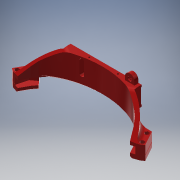
# Autodesk Inventor part: clamp_r
Saved by Autodesk Inventor 2017 (Build 210142000, 142)
## iProperties
Created: 2016-11-21
Part Number: clamp_r
Material: PC/ABS Plastic
Document SubType Name: Modeling
Designer: Ali
Density: 0.357273 g/cm^3
Appearance: Smooth - Red
Author: Ali
Autodesk Inventor part; units mm, degrees
sketch "Sketch1" plane through (0, 0, 0) normal (0, 0, 1) x (1, 0, 0)
  arc A0 (-5.3802, 56.637) -> (-102.6346, 44.8571) centre (-44.3802, -28.7347) ccw projected
  arc A1 (-102.6346, 44.8571) -> (-108.3066, 14.3732) centre (55.6325, -0.3603) ccw projected
  line L0 (-108.3066, 14.3732) -> (-107.3533, 6.1304) projected
  line L1 (-107.3533, 6.1304) -> (-107.3505, 6.0507) projected
  arc A2 (-107.3505, 6.0507) -> (-89.5835, -54.6922) centre (20.8962, 10.5923) ccw projected
  arc A3 (-89.5835, -54.6922) -> (-67.6974, -85.6874) centre (112.0298, 64.4449) ccw projected
  line L2 (-67.6974, -85.6874) -> (-66.8062, -86.7543) projected
  arc A4 (-66.8062, -86.7543) -> (-66.6302, -85.4767) centre (-71.3562, -85.4767) ccw projected
  arc A5 (-66.6302, -85.4767) -> (-74.3323, -73.8524) centre (-117.1754, -110.6039) ccw projected
  line L3 (-88.3802, -53.9767) -> (-74.3323, -73.8524) projected
  arc A6 (-105.1302, -3.9767) -> (-88.3802, -53.9767) centre (19.6205, 10.0092) ccw projected
  arc A7 (-104.1051, 25.3968) -> (-105.1302, -3.9767) centre (-5.1046, 7.2372) ccw projected
  spline S0 degree 4 poles (-44.3802, 62.2233) (-60.9817, 62.2233) (-84.9184, 55.4182) (-96.719, 46.0233) (-101.8787, 37.5346) (-104.1051, 25.3968) knots 1 1 1 1 1 2 3 3 3 3 3 projected
  spline S1 degree 4 poles (-44.3802, 62.2233) (-27.7787, 62.2233) (-3.8419, 55.4182) (7.9586, 46.0233) (13.1183, 37.5346) (15.3447, 25.3968) knots 1 1 1 1 1 2 3 3 3 3 3 projected
  arc A8 (16.3698, -3.9767) -> (15.3447, 25.3968) centre (-83.6558, 7.2372) ccw projected
  arc A9 (-0.3802, -53.9767) -> (16.3698, -3.9767) centre (-108.3809, 10.0092) ccw projected
  line L4 (-0.3802, -53.9767) -> (-14.428, -73.8524) projected
  arc A10 (-14.428, -73.8524) -> (-22.1302, -85.4767) centre (28.415, -110.6039) ccw projected
  arc A11 (-22.1302, -85.4767) -> (-21.9542, -86.7543) centre (-17.4041, -85.4767) ccw projected
  line L5 (-21.9542, -86.7543) -> (-21.063, -85.6874) projected
  arc A12 (-21.063, -85.6874) -> (0.8231, -54.6922) centre (-200.7901, 64.4449) ccw projected
  arc A13 (0.8231, -54.6922) -> (18.5901, 6.0507) centre (-109.6566, 10.5923) ccw projected
  line L6 (18.5901, 6.0507) -> (18.593, 6.1304) projected
  line L7 (18.593, 6.1304) -> (19.5462, 14.3732) projected
  arc A14 (19.5462, 14.3732) -> (13.8743, 44.8571) centre (-144.3928, -0.3603) ccw projected
  arc A15 (13.8743, 44.8571) -> (6.6198, 50.0583) centre (-44.3802, -28.7347) ccw projected
  line L8 (6.6198, 61.5233) -> (6.6198, 50.0583) projected
  line L9 (-5.3802, 61.5233) -> (6.6198, 61.5233) projected
  line L10 (-5.3802, 56.637) -> (-5.3802, 61.5233) projected
  line L11 (14.5194, 32.9809) -> (9.6506, 41.7615)
  line L12 (10.1861, 51.0026) -> (12.6488, 53.6391)
  line L13 (12.6488, 53.6391) -> (16.7857, 53.6391)
  line L14 (16.7857, 53.6391) -> (25.5146, 37.8973)
  line L15 (22.0832, 35.5866) -> (14.5194, 32.9809)
  line L16 (22.0832, 35.5866) -> (25.5146, 37.8973)
  line L17 (22.0832, 35.5866) -> (12.6488, 53.6391) construction
  line L18 (9.6506, 41.7615) -> (6.0073, 46.5287)
  line L19 (6.0073, 46.5287) -> (10.1861, 51.0026)
  line L20 (16.6197, 32.5233) -> (16.8713, 18.1048) projected
  line L21 (16.8878, 32.528) -> (16.6197, 32.5233) projected
  line L22 (16.8878, 32.528) -> (18.6194, 32.5582) projected
  line L23 (18.871, 18.1397) -> (18.6194, 32.5582) projected
  line L24 (18.871, 18.1397) -> (16.8713, 18.1048) projected
  line L25 (6.0073, 46.5287) -> (14.5194, 32.9809) construction
  point P0 (0, 0)
  dimension "d1" = 8
  dimension "d2" = 12
  dimension "d5" = 18
  dimension "d8" = 100
  dimension "d9" = 16
  dimension "d10" = 6
  constraints: 21 end point, 1 collinear, 1 equal length, 1 horizontal, 1 other
  measures "d1" distance of L15.start L11.start
  measures "d2" distance between parallel lines of L11 L14
  measures "d5" distance of L13.end L14.end
  measures "d8" angle of L15 L11
  measures "d9" distance of L18.end L11.start
  measures "d10" distance of L11.end L18.end
extrude "Extrusion1" add sketch "Sketch1" along normal blind 3 contours L19 L12 L13 L14 L16 L15 A14 A15 | A15 A14 L15 L11 L18 L19
sketch "Sketch2" plane through (0, 0, 0) normal (0, 0, -1) x (-1, 0, 0)
  line L0 (-14.5194, 32.9809) -> (-9.6506, 41.7615) projected
  line L1 (-9.6506, 41.7615) -> (-6.0073, 46.5287) projected
  line L2 (-6.0073, 46.5287) -> (-12.6488, 53.6391) projected
  line L3 (-12.6488, 53.6391) -> (-16.7857, 53.6391) projected
  line L4 (-16.7857, 53.6391) -> (-25.5146, 37.8973) projected
  line L5 (-25.5146, 37.8973) -> (-22.0832, 35.5866) projected
  line L6 (-22.0832, 35.5866) -> (-14.5194, 32.9809) projected
  line L7 (-6.0073, 46.5287) -> (-12.6488, 53.6391) projected
  line L8 (-12.6488, 53.6391) -> (-16.7857, 53.6391) projected
  line L9 (-9.328, 50.0839) -> (-12.6488, 53.6391)
  line L10 (-22.0832, 35.5866) -> (-14.5194, 32.9809) projected
  line L11 (-18.7662, 34.4439) -> (-22.0832, 35.5866)
  line L12 (-18.7662, 34.4439) -> (-15.745, 46.1362)
  line L13 (-12.6488, 53.6391) -> (-6.0073, 46.5287) projected
  line L14 (-9.7584, 50.5447) -> (-15.745, 46.1362)
  point P0 (0, 0)
  constraints: 8 end point, 2 point on line, 1 collinear, 1 midpoint
extrude "Extrusion2" add sketch "Sketch2" along normal blind 6.5 contours L6 L5 L4 L3 L2 L14 L12
sketch "Sketch3" plane through (0, 0, -6.5) normal (0, 0, -1) x (-1, 0, 0)
  line L0 (-9.6506, 41.7615) -> (-14.5194, 32.9809) projected
  line L1 (-14.5194, 32.9809) -> (-22.0832, 35.5866) projected
  line L2 (-22.0832, 35.5866) -> (-25.5146, 37.8973) projected
  line L3 (-25.5146, 37.8973) -> (-16.7857, 53.6391) projected
  line L4 (-16.7857, 53.6391) -> (-12.6488, 53.6391) projected
  line L5 (-12.6488, 53.6391) -> (-6.0073, 46.5287) projected
  line L6 (-6.0073, 46.5287) -> (-9.6506, 41.7615) projected
  point P0 (0, 0)
extrude "Extrusion3" add sketch "Sketch3" along normal blind 5 separate body
chamfer "Chamfer1" distance 1.5 angle 45 2 edges at (12.085, 37.3712, -11.5) (7.8289, 44.1451, -11.5)
sketch "Sketch4" plane through (0, 0, -11.5) normal (0, 0, -1) x (-1, 0, 0)
  line L0 (-7.0457, 47.6404) -> (-10.9091, 42.585) projected
  line L1 (-7.0457, 47.6404) -> (-12.6488, 53.6391) projected
  line L2 (-12.6488, 53.6391) -> (-16.7857, 53.6391) projected
  line L3 (-16.7857, 53.6391) -> (-25.5146, 37.8973) projected
  line L4 (-25.5146, 37.8973) -> (-22.0832, 35.5866) projected
  line L5 (-22.0832, 35.5866) -> (-15.9595, 33.477) projected
  line L6 (-10.9091, 42.585) -> (-15.9595, 33.477) projected
  point P0 (0, 0)
  point P1 (-15.5734, 49.6391)
  point P2 (-21.3927, 39.1446)
  dimension "d19" = 12
  dimension "d20" = 4
  dimension "d21" = 3
  dimension "d22" = 3
  measures "d19" distance of point (-21.393, 39.145) point (-15.573, 49.639)
  measures "d20" distance from line of L2 point (-15.573, 49.639)
  measures "d21" distance from line of L3 point (-15.573, 49.639)
  measures "d22" distance from line of point (-21.393, 39.145) L3
hole "Hole1" at (15.5734, 49.6391, -11.5) at (21.3927, 39.1446, -11.5) direction (0, 0, 1) diameter 2.2 end through all bodies 2
sketch "Sketch5" plane through (0, 0, -6.5) normal (0, 0, -1) x (-1, 0, 0)
  circle A0 centre (-21.3927, 39.1446) radius 1.1 projected
  circle A1 centre (-15.5734, 49.6391) radius 1.1 projected
  point P0 (0, 0)
hole "Hole2" at (21.3927, 39.1446, -6.5) at (15.5734, 49.6391, -6.5) direction (0, 0, 1) diameter 2.2 end through all bodies 1
ref_plane "Work Plane1" through (0, 0, 0) normal (0, 0, 1) x (1, 0, 0)
sketch "Sketch6" plane through (0, 0, 0) normal (0, 0, 1) x (1, 0, 0)
  arc A0 (-5.3802, 56.637) -> (-102.6346, 44.8571) centre (-44.3802, -28.7347) ccw projected
  arc A1 (-102.6346, 44.8571) -> (-108.3066, 14.3732) centre (55.6325, -0.3603) ccw projected
  line L0 (-108.3066, 14.3732) -> (-107.3533, 6.1304) projected
  line L1 (-107.3533, 6.1304) -> (-107.3505, 6.0507) projected
  arc A2 (-107.3505, 6.0507) -> (-89.5835, -54.6922) centre (20.8962, 10.5923) ccw projected
  arc A3 (-89.5835, -54.6922) -> (-67.6974, -85.6874) centre (112.0298, 64.4449) ccw projected
  line L2 (-67.6974, -85.6874) -> (-66.8062, -86.7543) projected
  arc A4 (-66.8062, -86.7543) -> (-66.6302, -85.4767) centre (-71.3562, -85.4767) ccw projected
  arc A5 (-66.6302, -85.4767) -> (-74.3323, -73.8524) centre (-117.1754, -110.6039) ccw projected
  line L3 (-88.3802, -53.9767) -> (-74.3323, -73.8524) projected
  arc A6 (-105.1302, -3.9767) -> (-88.3802, -53.9767) centre (19.6205, 10.0092) ccw projected
  arc A7 (-104.1051, 25.3968) -> (-105.1302, -3.9767) centre (-5.1046, 7.2372) ccw projected
  spline S0 degree 4 poles (-44.3802, 62.2233) (-60.9817, 62.2233) (-84.9184, 55.4182) (-96.719, 46.0233) (-101.8787, 37.5346) (-104.1051, 25.3968) knots 1 1 1 1 1 2 3 3 3 3 3 projected
  spline S1 degree 4 poles (-44.3802, 62.2233) (-27.7787, 62.2233) (-3.8419, 55.4182) (7.9586, 46.0233) (13.1183, 37.5346) (15.3447, 25.3968) knots 1 1 1 1 1 2 3 3 3 3 3 projected
  arc A8 (16.3698, -3.9767) -> (15.3447, 25.3968) centre (-83.6558, 7.2372) ccw projected
  arc A9 (-0.3802, -53.9767) -> (16.3698, -3.9767) centre (-108.3809, 10.0092) ccw projected
  line L4 (-0.3802, -53.9767) -> (-14.428, -73.8524) projected
  arc A10 (-14.428, -73.8524) -> (-22.1302, -85.4767) centre (28.415, -110.6039) ccw projected
  arc A11 (-22.1302, -85.4767) -> (-21.9542, -86.7543) centre (-17.4041, -85.4767) ccw projected
  line L5 (-21.9542, -86.7543) -> (-21.063, -85.6874) projected
  arc A12 (-21.063, -85.6874) -> (0.8231, -54.6922) centre (-200.7901, 64.4449) ccw projected
  arc A13 (0.8231, -54.6922) -> (18.5901, 6.0507) centre (-109.6566, 10.5923) ccw projected
  line L6 (18.5901, 6.0507) -> (18.593, 6.1304) projected
  line L7 (18.593, 6.1304) -> (19.5462, 14.3732) projected
  arc A14 (19.5462, 14.3732) -> (13.8743, 44.8571) centre (-144.3928, -0.3603) ccw projected
  arc A15 (13.8743, 44.8571) -> (6.6198, 50.0583) centre (-44.3802, -28.7347) ccw projected
  line L8 (6.6198, 61.5233) -> (6.6198, 50.0583) projected
  line L9 (-5.3802, 61.5233) -> (6.6198, 61.5233) projected
  line L10 (-5.3802, 56.637) -> (-5.3802, 61.5233) projected
  line L11 (-44.3802, 62.2233) -> (-44.3802, 62.8011) construction
  circle A16 centre (21.3927, 39.1446) radius 1.1 projected
  circle A17 centre (15.5734, 49.6391) radius 1.1 projected
  line L12 (9.6506, 41.7615) -> (14.5194, 32.9809) projected
  line L13 (14.5194, 32.9809) -> (22.0832, 35.5866) projected
  line L14 (22.0832, 35.5866) -> (25.5146, 37.8973) projected
  line L15 (25.5146, 37.8973) -> (16.7857, 53.6391) projected
  line L16 (16.7857, 53.6391) -> (12.6488, 53.6391) projected
  line L17 (12.6488, 53.6391) -> (6.0073, 46.5287) projected
  line L18 (6.0073, 46.5287) -> (9.6506, 41.7615) projected
  spline S2 degree 3 poles (6.0073, 46.5287) (-6.3628, 57.3321) (-25.7237, 62.8011) (-44.3802, 62.8011) knots 0 0 0 0 1 1 1 1
  line L19 (-44.3802, 62.8011) -> (-44.3802, 66.8011)
  line L20 (16.7857, 53.6391) -> (12.6488, 53.6391) projected
  line L21 (12.6488, 53.6391) -> (0.9642, 53.6391) construction
  line L22 (0.9642, 53.6391) -> (-13.174, 64.4449) construction
  line L23 (-13.174, 64.4449) -> (-32.5316, 66.8011) construction
  line L24 (-32.5316, 66.8011) -> (-44.3802, 66.8011) construction
  spline S3 degree 4 poles (12.6488, 53.6391) (0.9642, 53.6391) (-13.174, 64.4449) (-32.5316, 66.8011) (-44.3802, 66.8011) knots 1 1 1 1 1 2 2 2 2 2
  point P0 (0, 0)
  point P1 (-15.8694, 58.4105)
  dimension "d38" = 4
  constraints: 4 end point, 4 vertical, 1 collinear, 6 other
  measures "d38" distance of L11.end L19.end
extrude "Extrusion4" add sketch "Sketch6" along normal up to surface (3 mm away) contours L10 S3 L8 A15 L17 S2 L19 A0 | A0 L19 S3 L10 | S3 L17 A15 L8 bodies 1
sketch "Sketch7" plane through (0, 0, 3) normal (0, 0, 1) x (1, 0, 0)
  circle A0 centre (21.3927, 39.1446) radius 1.1 projected
  circle A1 centre (15.5734, 49.6391) radius 1.1 projected
  line L0 (9.6506, 41.7615) -> (14.5194, 32.9809) projected
  line L1 (14.5194, 32.9809) -> (22.0832, 35.5866) projected
  line L2 (22.0832, 35.5866) -> (25.5146, 37.8973) projected
  line L3 (25.5146, 37.8973) -> (16.7857, 53.6391) projected
  line L4 (16.7857, 53.6391) -> (12.6488, 53.6391) projected
  spline S0 degree 4 poles (-44.3802, 66.8011) (-32.5316, 66.8011) (-13.174, 64.4449) (0.9642, 53.6391) (12.6488, 53.6391) knots 0 0 0 0 0 1 1 1 1 1 projected
  line L5 (-44.3802, 62.8011) -> (-44.3802, 66.8011) projected
  spline S1 degree 3 poles (6.0073, 46.5287) (-6.3628, 57.3321) (-25.7237, 62.8011) (-44.3802, 62.8011) knots 0 0 0 0 1 1 1 1 projected
  line L6 (6.0073, 46.5287) -> (9.6506, 41.7615) projected
  line L7 (14.5194, 32.9809) -> (22.0832, 35.5866) projected
  arc A2 (18.7914, 34.4526) -> (-7.163, 59.1735) centre (-22.4149, 17.1754) ccw
  line L8 (-7.163, 59.1735) -> (-7.163, 66.8011)
  line L9 (-44.3802, 66.8011) -> (-44.3802, 62.8011) projected
  line L10 (-7.163, 66.8011) -> (-44.3802, 66.8011)
  point P0 (0, 0)
  constraints: 4 end point, 2 point on circle, 1 centre point, 1 perpendicular, 1 point on line, 1 vertical, 4 other
extrude "Extrusion5" add sketch "Sketch7" along normal blind 24 contours L6 S1 L5 S0 A2 L1 L0 | S0 L10 L8 bodies 1
sketch "Sketch13" plane through (0, 0, 3) normal (0, 0, -1) x (-1, 0, 0)
  spline S0 degree 4 poles (44.3802, 66.8011) (36.9623, 66.8011) (26.6014, 65.8776) (16.4206, 62.5354) (7.163, 59.1735) knots 0 0 0 0 0 1 1 1 1 1 projected
  line L0 (7.163, 66.8011) -> (44.3802, 66.8011) projected
  line L1 (7.163, 59.1735) -> (7.163, 66.8011) projected
  point P0 (0, 0)
  constraints: 1 other
extrude "Extrusion10" cut sketch "Sketch13" against normal blind 4 bodies 1
sketch "Sketch8" plane through (16.7857, 53.6391, 3) normal (0.8745473, 0.4849403, 0) x (0, 0, -1)
  line L0 (0, -17.7522) -> (-24, -17.7522) projected
  line L1 (-24, 16.4538) -> (-24, 23.1244) projected
  line L2 (0, -17.7522) -> (-24, 16.4538)
  line L3 (-24, -17.7522) -> (-24, 16.4538)
  point P0 (3, -38.7699)
  constraints: 4 end point
extrude "Extrusion6" cut sketch "Sketch8" against normal through all bodies 1
sketch "Sketch15" plane through (0, 0, 3) normal (0, 0, 1) x (1, 0, 0)
  line L0 (25.5146, 37.8973) -> (16.7857, 53.6391) projected
  line L1 (16.7857, 53.6391) -> (12.6488, 53.6391) projected
  arc A0 (18.7914, 34.4526) -> (-7.163, 59.1735) centre (-22.4149, 17.1754) ccw projected
  line L2 (18.7914, 34.4526) -> (22.0832, 35.5866) projected
  line L3 (22.0832, 35.5866) -> (25.5146, 37.8973) projected
  circle A1 centre (21.3927, 39.1446) radius 1.1 projected
  circle A2 centre (15.5734, 49.6391) radius 1.1 projected
  line L4 (19.0547, 39.185) -> (20.2587, 41.1895)
  line L5 (20.2587, 41.1895) -> (22.5967, 41.149)
  line L6 (22.5967, 41.149) -> (23.7306, 39.1041)
  line L7 (23.7306, 39.1041) -> (22.5266, 37.0996)
  line L8 (22.5266, 37.0996) -> (20.1887, 37.1401)
  line L9 (20.1887, 37.1401) -> (19.0547, 39.185)
  circle A3 centre (15.5734, 49.6391) radius 1.1 projected
  line L10 (13.2355, 49.6796) -> (14.4395, 51.6841)
  line L11 (14.4395, 51.6841) -> (16.7774, 51.6436)
  line L12 (16.7774, 51.6436) -> (17.9113, 49.5987)
  line L13 (17.9113, 49.5987) -> (16.7073, 47.5942)
  line L14 (16.7073, 47.5942) -> (14.3694, 47.6347)
  line L15 (14.3694, 47.6347) -> (13.2355, 49.6796)
  line L16 (25.5146, 37.8973) -> (16.7857, 53.6391) projected
  point P0 (0, 0)
  dimension "d89" = 4.05
  dimension "d90" = 4.05
  constraints: 24 end point, 2 coincident, 2 parallel, 27 other
  measures "d89" distance between parallel lines of L4 L7
  measures "d90" distance between parallel lines of L13 L10
extrude "Extrusion11" cut sketch "Sketch15" against normal blind 4 bodies 1
mirror "Mirror1" about plane through (-44.3802, 66.8011, 0) normal (-1, 0, 0) of "Extrusion5", "Extrusion6", "Extrusion1", "Hole2", "Extrusion2", "Extrusion4", "Extrusion10", "Extrusion11" bodies 1
sketch "Sketch9" plane through (-7.163, 66.8011, 27) normal (0, 1, 0) x (1, 0, 0)
  line L0 (41.7828, 2) -> (-116.2172, 2)
  line L1 (-116.2172, 2) -> (-116.2172, 18)
  line L2 (-116.2172, 18) -> (41.7828, 18)
  line L3 (41.7828, 18) -> (41.7828, 2)
  line L4 (-74.4343, 20) -> (-74.4343, 0) projected
  line L5 (0, 0) -> (-74.4343, 0) projected
  line L6 (0, 20) -> (0, 0) projected
  line L7 (-37.2172, 24) -> (-37.2172, 0) construction
  line L8 (-74.4343, 24) -> (-37.2172, 24) projected
  line L9 (-56.7172, 16.2) -> (-56.7172, 3.8) construction
  line L10 (0, 20) -> (-37.2172, 20) projected
  line L11 (-37.2172, 20) -> (-74.4343, 20) projected
  point P0 (7.163, 27)
  point P1 (-37.2172, 2)
  dimension "d45" = 158
  dimension "d46" = 16
  dimension "d47" = 1.8
  dimension "d48" = 1.8
  dimension "d49" = 59.5
  dimension "d62" = 2
  constraints: 10 end point, 2 parallel, 1 horizontal, 1 midpoint, 1 perpendicular, 1 point on line, 1 vertical
  measures "d45" distance of L0.start L0.end
  measures "d46" distance of L0.end L1.end
  measures "d47" distance from line of L0 L9.end
  measures "d48" distance from line of L2 L9.start
  measures "d49" distance between parallel lines of L9 L1
  measures "d62" distance between parallel lines of L5 L0
hole "Hole3" at (-63.8802, 66.8011, 23.2) at (-63.8802, 66.8011, 10.8) direction (0, -1, 0) diameter 1.8 end through all bodies 1
ref_plane "Work Plane2" through (-7.163, 56.5511, 27) normal (0, 1, 0) x (1, 0, 0)
sketch "Sketch10" plane through (-7.163, 56.5511, 27) normal (0, 1, 0) x (1, 0, 0)
  spline S0 degree 2 poles (-56.7172, 2.9) (-58.276, 2.9) (-57.4966, 4.25) (-56.7172, 5.6) (-55.9377, 4.25) (-55.1583, 2.9) (-56.7172, 2.9) knots 0 0 0 0.333333 0.333333 0.666667 0.666667 1 1 1 weights 1 0.5 1 0.5 1 0.5 1 projected
  spline S1 degree 2 poles (-56.7172, 15.3) (-58.276, 15.3) (-57.4966, 16.65) (-56.7172, 18) (-55.9377, 16.65) (-55.1583, 15.3) (-56.7172, 15.3) knots 0 0 0 0.333333 0.333333 0.666667 0.666667 1 1 1 weights 1 0.5 1 0.5 1 0.5 1 projected
  circle A0 centre (-56.7172, 3.8) radius 0.9 projected
  circle A1 centre (-56.7172, 3.8) radius 2
  circle A2 centre (-56.7172, 16.2) radius 0.9 projected
  circle A3 centre (-56.7172, 16.2) radius 2
  line L0 (-54.7172, 16.2) -> (-54.7172, 3.8)
  line L1 (-58.7172, 3.8) -> (-58.7172, 16.2)
  point P0 (7.163, 27)
  dimension "d58" = 4
  dimension "d59" = 4
  constraints: 4 end point, 4 point on circle, 2 centre point, 2 coincident, 2 tangent, 2 vertical, 4 other
  measures "d58" diameter of A1
  measures "d59" diameter of A3
extrude "Extrusion7" cut sketch "Sketch10" along normal blind 8.6 bodies 1
sketch "Sketch11" plane through (-7.163, 66.8011, 27) normal (0, 1, 0) x (1, 0, 0)
  circle A0 centre (-56.7172, 3.8) radius 0.9 projected
  circle A1 centre (-56.7172, 16.2) radius 0.9 projected
  line L0 (-74.4343, 20) -> (-74.4343, 0) projected
  line L1 (0, 0) -> (-74.4343, 0) projected
  line L2 (0, 20) -> (0, 0) projected
  line L3 (0, 20) -> (0, 0) projected
  line L4 (0, 2) -> (-74.4343, 2)
  line L5 (-74.4343, 20) -> (-74.4343, 0) projected
  line L6 (-74.4343, 18) -> (0, 18)
  line L7 (-37.2172, 20) -> (-74.4343, 20) projected
  line L8 (0, 20) -> (-37.2172, 20) projected
  point P0 (7.163, 27)
  point P1 (0, 24)
  point P2 (-74.4343, 24)
  dimension "d63" = 2
  dimension "d78" = 16
  constraints: 4 end point, 4 point on line, 1 horizontal, 1 parallel
  measures "d63" distance between parallel lines of L1 L4
  measures "d78" distance between parallel lines of L4 L6
extrude "Extrusion8" cut sketch "Sketch11" against normal blind 0.5 contours A0 | A1 | L6 L2 L4 L0 bodies 1
sketch "Sketch12" plane through (-7.163, 66.3011, 27) normal (0, 1, 0) x (1, 0, 0)
  arc A0 (-12.9987, -3.5935) -> (-2.9987, -3.5935) centre (-7.9987, -3.5935) ccw projected
  line L0 (-2.9987, 0) -> (-2.9987, -3.5935) projected
  line L1 (-12.9987, -3.5935) -> (-12.9987, 0) projected
  line L2 (-2.9987, 0) -> (-12.9987, 0)
  point P0 (7.163, 27)
  constraints: 2 end point
extrude "Extrusion9" add sketch "Sketch12" against normal blind 4 bodies 1
hole "Hole4" at (-15.1617, 62.3011, 30.5935) direction (0, 1, 0) diameter 2.2 end through all counterbore diameter 4.5 counterbore depth 1.5 bodies 1
sketch "Sketch17" plane through (0, 0, -6.5) normal (0, 0, 1) x (1, 0, 0)
  circle A0 centre (15.5734, 49.6391) radius 1.1 projected
  circle A1 centre (21.3927, 39.1446) radius 1.1 projected
  line L0 (9.6506, 41.7615) -> (14.5194, 32.9809) projected
  line L1 (14.5194, 32.9809) -> (22.0832, 35.5866) projected
  line L2 (22.0832, 35.5866) -> (25.5146, 37.8973) projected
  line L3 (25.5146, 37.8973) -> (16.7857, 53.6391) projected
  line L4 (16.7857, 53.6391) -> (12.6488, 53.6391) projected
  line L5 (12.6488, 53.6391) -> (6.0073, 46.5287) projected
  line L6 (6.0073, 46.5287) -> (9.6506, 41.7615) projected
  line L7 (18.7662, 34.4439) -> (15.745, 46.1362) projected
  line L8 (15.745, 46.1362) -> (9.7584, 50.5447) projected
  point P0 (0, 0)
extrude "Extrusion13" cut sketch "Sketch17" against normal blind 0.65 contours L6 L5 L8 L7 L1 L0 bodies 2
chamfer "Chamfer4" distance 1.2 angle 45 2 edges at (21.3927, 38.0446, -11.5) (15.5734, 48.5391, -11.5)
ref_plane "Work Plane3" through (-44.3802, 62.8011, 27) normal (1, 0, 0) x (0, 1, 0)
mirror "Mirror2" about plane through (-44.3802, 62.8011, 27) normal (1, 0, 0) bodies 2
sketch "Sketch14" plane through (0, 0, 27) normal (0, 0, 1) x (1, 0, 0)
  line L0 (-20.1617, 62.3011) -> (-20.1617, 66.3011) projected
  line L1 (-20.1617, 66.3011) -> (-10.1617, 66.3011) projected
  line L2 (-10.1617, 66.3011) -> (-10.1617, 62.3011) projected
  line L3 (-10.1617, 62.3011) -> (-20.1617, 62.3011) projected
  line L4 (-81.5973, 59.1735) -> (-77.3415, 56.8136) projected
  line L5 (-11.4189, 56.8136) -> (-7.163, 59.1735) projected
  line L6 (-7.163, 59.1735) -> (-7.163, 66.8011) projected
  line L7 (-7.163, 66.8011) -> (-81.5973, 66.8011) projected
  line L8 (-81.5973, 59.1735) -> (-81.5973, 66.8011) projected
  line L9 (-29.3802, 64.2297) -> (-59.3802, 64.2297) construction
  line L10 (-44.3802, 62.8011) -> (-44.3802, 53.9631) construction
  point P0 (0, 0)
  point P1 (-44.3802, 64.2297)
  dimension "d81" = 30
  constraints: 4 end point, 1 midpoint, 1 parallel, 1 point on line, 1 vertical, 2 other
  measures "d81" distance of L9.end L9.start
hole "Hole5" at (-29.3802, 64.2297, 27) at (-59.3802, 64.2297, 27) direction (0, 0, -1) diameter 1.8 depth 8 tip angle 118 bodies 1
fillet "Fillet1" radius 12 2 edges at (-79.4694, 57.9935, 27) (-9.291, 57.9935, 27)
fillet "Fillet2" radius 4 2 edges at (8.4017, 49.5296, 3) (-97.1621, 49.5296, 3)
chamfer "Chamfer3" distance 2 angle 45 2 edges at (-71.9313, 58.7162, 0) (-16.8291, 58.7162, 0)
equation "\"d90\" = d89"
